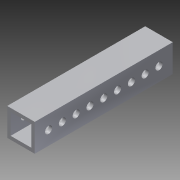
# Autodesk Inventor part: Chassis V1.500 Part8
Saved by Autodesk Inventor 2013 (Build 170138000, 138)
## iProperties
Created: 2013-01-18
Part Number: Chassis V1.500 Part8
Material: Aluminum 6061
Document SubType Name: Modeling
Designer: Moses
Mass: 94.1973 g
Surface Area: 231.188 cm^2
Volume: 34.7592 cm^3
Density: 2.71 g/cm^3
Author: Moses
Autodesk Inventor part; units mm, degrees
ref_plane "YZ Plane" through (0, 0, 0) normal (1, 0, 0) x (0, 1, 0)
ref_plane "XZ Plane" through (0, 0, 0) normal (0, 1, 0) x (-1, 0, 0)
ref_plane "XY Plane" through (0, 0, 0) normal (0, 0, 1) x (1, 0, 0)
sketch "Sketch1" plane through (0, 0, 0) normal (0, 0, 1) x (1, 0, 0)
  line L0 (0, 0) -> (25.4, 0)
  line L1 (25.4, 0) -> (25.4, 25.4)
  line L2 (25.4, 25.4) -> (0, 25.4)
  line L3 (0, 25.4) -> (0, 0)
  line L4 (3.175, 22.225) -> (22.225, 22.225)
  line L5 (22.225, 22.225) -> (22.225, 3.175)
  line L6 (22.225, 3.175) -> (3.175, 3.175)
  line L7 (3.175, 3.175) -> (3.175, 22.225)
  dimension "d0" = 25.4
  dimension "d1" = 25.4
  dimension "d2" = 3.175
  constraints: 16 end point, 4 parallel, 2 perpendicular, 1 horizontal, 3 other
  measures "d0" distance of L2.end L1.end
  measures "d1" distance of L1.end L0.end
  measures "d2" distance between parallel lines of L1 L5
extrude "Extrusion1" add sketch "Sketch1" along normal blind 127
sketch "Sketch2" plane through (25.4, 0, 0) normal (1, 0, 0) x (0, 0, -1)
  line L0 (0, 0) -> (0, 25.4) projected
  line L1 (-127, 0) -> (-127, 25.4) projected
  line L2 (0, 0) -> (-127, 0) projected
  line L3 (-127, 12.7) -> (-114.3, 12.7) construction
  line L4 (0, 12.7) -> (-12.7, 12.7) construction
  circle A0 centre (-114.3, 12.7) radius 3.302
  line L5 (0, 25.4) -> (-127, 25.4) projected
  line L6 (-114.3, 12.7) -> (-12.7, 12.7) construction
  circle A1 centre (-101.6, 12.7) radius 3.302
  circle A2 centre (-88.9, 12.7) radius 3.302
  circle A3 centre (-76.2, 12.7) radius 3.302
  circle A4 centre (-63.5, 12.7) radius 3.302
  circle A5 centre (-50.8, 12.7) radius 3.302
  circle A6 centre (-38.1, 12.7) radius 3.302
  circle A7 centre (-25.4, 12.7) radius 3.302
  circle A8 centre (-12.7, 12.7) radius 3.302
  dimension "d5" = 12.7
  dimension "d7" = 6.604
  dimension "d13" = 127
  dimension "d16" = 12.7
  constraints: 9 centre point, 6 end point, 2 coincident, 2 midpoint, 2 parallel, 1 collinear, 1 horizontal, 16 other
  measures "d5" distance of L3.start L3.end
  measures "d7" diameter of A0
  measures "d13" distance of L0.end L1.end
  measures "d16" distance of L6.start A1.centre
extrude "Extrusion2" cut sketch "Sketch2" against normal through all contours A0 | A1 | A2 | A3 | A4 | A5 | A6 | A7 | A8
equation "\"d16\" = -0.25 * d5 + 0.125 * d13"
body "Solid1"
